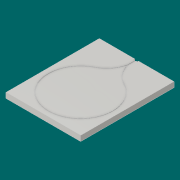
# Autodesk Inventor part: Scintillator Tile
Saved by Autodesk Inventor 2016 (Build 200138000, 138)
## iProperties
Created: 2015-08-14
Part Number: Scintillator Tile
Material: ABS Plastic
Document SubType Name: Modeling
Designer: Cosmic
Density: 1.06 g/cm^3
Appearance: Smooth - White
Author: Cosmic
Autodesk Inventor part; units mm, degrees
ref_plane "YZ Plane" through (0, 0, 0) normal (1, 0, 0) x (0, 1, 0)
ref_plane "XZ Plane" through (0, 0, 0) normal (0, 1, 0) x (-1, 0, 0)
ref_plane "XY Plane" through (0, 0, 0) normal (0, 0, 1) x (1, 0, 0)
sketch "Sketch1" plane through (0, 0, 0) normal (0, 0, 1) x (1, 0, 0)
  line L0 (-70, -87.5) -> (70, -87.5)
  line L1 (70, -87.5) -> (70, 87.5)
  line L2 (70, 87.5) -> (-70, 87.5)
  line L3 (-70, 87.5) -> (-70, -87.5)
  line L4 (-70, -87.5) -> (70, 87.5) construction
  line L5 (70, -87.5) -> (-70, 87.5) construction
  point P0 (0, 0)
  dimension "d0" = 140
  dimension "d1" = 175
  constraints: 12 end point, 2 midpoint, 2 parallel, 1 horizontal, 1 perpendicular
  measures "d0" distance of L2.end L1.end
  measures "d1" distance of L1.end L0.end
extrude "Extrusion1" add sketch "Sketch1" along normal blind 10
sketch "Sketch2" plane through (0, 0, 10) normal (0, 0, 1) x (1, 0, 0)
  line L0 (-70, -87.5) -> (70, -87.5) projected
  line L1 (70, -87.5) -> (70, 87.5) projected
  line L2 (70, 87.5) -> (-70, 87.5) projected
  line L3 (-70, 87.5) -> (-70, -87.5) projected
  line L4 (70, 87.5) -> (-70, 87.5) projected
  line L5 (-70, -87.5) -> (70, -87.5) projected
  line L6 (-5.4917, 87.5) -> (5.4917, 87.5)
  line L7 (-75.0628, -87.5) -> (-85.4917, -87.5)
  line L8 (50.6895, 87.5) -> (61.7911, 87.5)
  line L9 (-18.2089, -87.5) -> (-29.3105, -87.5)
  arc A0 (-27.0027, 36.0804) -> (27.0027, 36.0804) centre (0, -17.5) ccw
  arc A1 (-27.4977, 37.0627) -> (27.4977, 37.0627) centre (0, -17.5) ccw
  line L10 (-1, 87.5) -> (1, 87.5)
  line L11 (-1.1, 87.5) -> (1.1, 87.5)
  line L12 (1.1, 87.5) -> (1.1, 71.2827)
  line L13 (1.1, 66.8806) -> (-1.1, 66.8806)
  line L14 (-1.1, 71.2827) -> (-1.1, 87.5)
  arc A2 (1.1, 66.8806) -> (27.0027, 36.0804) centre (50, 81.713) ccw
  arc A3 (-27.4977, 37.0627) -> (-1.1, 71.2827) centre (-50, 81.713) ccw
  arc A4 (1.1, 71.2827) -> (27.4977, 37.0627) centre (50, 81.713) ccw
  arc A5 (-27.0027, 36.0804) -> (-1.1, 66.8806) centre (-50, 81.713) ccw
  line L15 (0, 87.5) -> (0, 81.713)
  line L16 (0, 71.1673) -> (0, -17.5)
  line L17 (-1.1, 87.5) -> (1.1, 87.5)
  point P0 (0, 66.8806)
  dimension "d4" = 120
  dimension "d5" = 1.1
  dimension "d23" = 2.2
  dimension "d26" = 70
  dimension "d27" = 70
  dimension "d28" = 140
  constraints: 24 end point, 12 point on circle, 8 point on line, 6 centre point, 5 horizontal, 4 parallel, 3 perpendicular, 2 midpoint, 17 other
  measures "d4" diameter of A0
  measures "d5" radial gap between concentric circles of A0 A1
  measures "d23" distance of L13.end L13.start
  measures "d26" distance from line of L0 L16.end
  measures "d27" distance from line of L3 L15.start
  measures "d28" distance between parallel lines of L3 L1
extrude "Extrusion6" cut sketch "Sketch2" against normal blind 1.1 contours L2 L12 A4 A1 A3 L14
sketch "Sketch3" plane through (0, 0, 10) normal (0, 0, 1) x (1, 0, 0)
  line L0 (-1.1, 71.2827) -> (-1.1, 87.5) projected
  line L1 (-1.1, 87.5) -> (-70, 87.5) projected
  line L2 (-70, 87.5) -> (-70, -87.5) projected
  line L3 (-70, -87.5) -> (70, -87.5) projected
  line L4 (70, -87.5) -> (70, 87.5) projected
  line L5 (70, 87.5) -> (1.1, 87.5) projected
  line L6 (1.1, 87.5) -> (1.1, 71.2827) projected
  arc A0 (1.1, 71.2827) -> (27.4977, 37.0627) centre (50, 81.713) ccw projected
  arc A1 (-27.4977, 37.0627) -> (27.4977, 37.0627) centre (0, -17.5) ccw projected
  arc A2 (-27.4977, 37.0627) -> (-1.1, 71.2827) centre (-50, 81.713) ccw projected
  line L7 (70, 87.5) -> (-70, 87.5) projected
  line L8 (-3.4, 87.5) -> (3.4, 87.5)
  line L9 (3.4, 87.5) -> (3.4, 85.3)
  line L10 (3.4, 85.3) -> (-3.4, 85.3)
  line L11 (-3.4, 85.3) -> (-3.4, 87.5)
  point P0 (0, 0)
  point P1 (0, 87.5)
  dimension "d31" = 2.2
  dimension "d32" = 6.8
  dimension "d36" = 1.1
  dimension "d37" = 1.1
  constraints: 8 end point, 2 midpoint, 2 parallel, 1 horizontal, 1 perpendicular, 1 point on line
  measures "d31" distance of L8.end L9.end
  measures "d32" distance between parallel lines of L9 L11
extrude "Extrusion7" cut sketch "Sketch3" against normal blind 6.15 contours L10 L11 L1 L0 | L0 L7 L6 L10 | L6 L5 L9 L10
equation "\"d23\" = 2 * d5"
equation "\"d27\" = 0.5 * d28"
equation "\"d29\" = d5"
equation "\"d21\" = d5"
equation "\"d22\" = d5"
body "Solid1"
